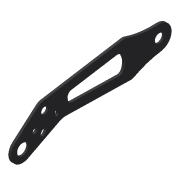
# Autodesk Inventor part: UPPER_LEG_OUTER_FRAME
Saved by Autodesk Inventor 2019.4 (Build 234330000, 330)
## iProperties
Created: 2019-11-12
Part Number: UPPER_LEG_OUTER_FRAME
Material: 一般
Document SubType Name: Modeling
Designer: y6tada
Density: 1 g/cm^3
Appearance: Black 80
Mass: 5.99749 g
Surface Area: 71.6947 cm^2
Volume: 5.99749 cm^3
Author: y6tada
Autodesk Inventor part; units mm, degrees
ref_plane "YZ Plane" through (0, 0, 0) normal (1, 0, 0) x (0, 1, 0)
ref_plane "XZ Plane" through (0, 0, 0) normal (0, 1, 0) x (-1, 0, 0)
ref_plane "XY Plane" through (0, 0, 0) normal (0, 0, 1) x (1, 0, 0)
sketch "スケッチ1" plane through (0, 0, 0) normal (1, 0, 0) x (0, 1, 0)
  line L0 (0, 0) -> (-25, 122.4745) construction
  line L1 (0, 189.3993) -> (0, 0) construction
  line L2 (1.3896, 108.1627) -> (-17.0322, 129.3894)
  arc A0 (-17.0322, 129.3894) -> (-34.3718, 117.6297) centre (-25, 122.4745) ccw
  arc A1 (3.2791, 104.1358) -> (1.3896, 108.1627) centre (-4.7732, 102.8143) ccw
  arc A2 (-17.7874, 128.734) -> (-30.0598, 114.375) centre (-25, 122.4745) ccw construction
  circle A3 centre (-4.7732, 102.8143) radius 7.16 construction
  line L3 (2.2923, 103.9738) -> (18.8479, 3.0931) construction
  line L4 (0.6344, 107.5073) -> (-17.7874, 128.734) construction
  line L5 (-30.0598, 114.375) -> (-18.9414, 107.4293) construction
  line L6 (-16.9441, 103.7364) -> (-19.0959, 0.3976) construction
  arc A4 (-16.9441, 103.7364) -> (-18.9414, 107.4293) centre (-21.1932, 103.8249) ccw construction
  circle A5 centre (-21.1932, 103.8249) radius 4 construction
  arc A6 (-21.8382, 104.2725) -> (-20.5116, 103.4352) centre (-16.3894, 111.4356) ccw construction
  arc A7 (-23.0793, 102.6409) -> (-21.4505, 101.6128) centre (-16.3894, 111.4356) ccw
  arc A8 (-21.4505, 101.6128) -> (-19.5726, 105.2575) centre (-20.5116, 103.4352) ccw
  arc A9 (-20.5971, 105.9041) -> (-23.0793, 102.6409) centre (-21.8382, 104.2725) ccw
  line L7 (-20.5116, 103.4352) -> (-16.3894, 111.4356) construction
  line L8 (-16.3894, 111.4356) -> (-21.8382, 104.2725) construction
  circle A10 centre (-16.3894, 111.4356) radius 2.05
  line L9 (-25, 122.4745) -> (-16.3894, 111.4356) construction
  arc A11 (14.8297, 29.3873) -> (10.9795, 0.6715) centre (85.8396, 5.2502) ccw
  arc A12 (-10.8792, -1.6259) -> (10.9795, 0.6715) centre (0, 0) ccw
  arc A13 (-10.8792, -1.6259) -> (-18.8693, 22.5646) centre (-85.0554, -12.7116) ccw
  line L10 (15.0698, 32.2899) -> (3.2791, 104.1358)
  line L11 (-18.3235, 85.5278) -> (-19.5731, 25.5116)
  line L12 (-16.3894, 111.4356) -> (-21.1932, 103.8249) construction
  arc A14 (-20.5971, 105.9041) -> (-19.5726, 105.2575) centre (-16.3894, 111.4356) ccw
  arc A15 (-13.6957, 91.6178) -> (-10.2953, 92.3867) centre (-16.3894, 111.4356) ccw construction
  line L13 (-10.2953, 92.3867) -> (-16.3894, 111.4356) construction
  line L14 (-13.6957, 91.6178) -> (-16.3894, 111.4356) construction
  arc A16 (-13.8371, 92.6583) -> (-10.6152, 93.3867) centre (-16.3894, 111.4356) ccw
  arc A17 (-13.5542, 90.5774) -> (-9.9753, 91.3866) centre (-16.3894, 111.4356) ccw
  arc A18 (-9.9753, 91.3866) -> (-10.6152, 93.3867) centre (-10.2953, 92.3867) ccw
  arc A19 (-13.8371, 92.6583) -> (-13.5542, 90.5774) centre (-13.6957, 91.6178) ccw
  line L15 (0, 0) -> (-9.0971, 86.5528) construction
  line L16 (-16.3894, 111.4356) -> (-11.9787, 91.928) construction
  arc A20 (-19.0959, 0.3976) -> (18.8479, 3.0931) centre (0, 0) ccw construction
  line L17 (-34.3718, 117.6297) -> (-18.7693, 87.4479)
  arc A21 (-18.3235, 85.5278) -> (-18.7693, 87.4479) centre (-22.3226, 85.611) ccw
  circle A22 centre (-21.1932, 103.8249) radius 5 construction
  arc A23 (14.8297, 29.3873) -> (15.0698, 32.2899) centre (9.149, 31.3183) ccw
  arc A24 (-19.5731, 25.5116) -> (-18.8693, 22.5646) centre (-13.5744, 25.3867) ccw
  circle A25 centre (-21.8382, 104.2725) radius 5 construction
  line L18 (10.9795, 0.6715) -> (0, 0) construction
  line L19 (0, 0) -> (-10.8792, -1.6259) construction
  line L20 (5.3923, 89.8056) -> (-23.9461, 86.722) construction
  line L21 (-15.4306, 104.3676) -> (-17.568, 1.7197) construction
  circle A26 centre (-13.6957, 91.6178) radius 2 construction
  line L22 (6.0142, 38.0699) -> (-0.6771, 78.8428)
  line L23 (-10.4767, 78.0835) -> (-11.3537, 35.9665)
  line L24 (-5.0424, 82.1731) -> (-6.8957, 81.9783)
  circle A27 centre (-3.7775, 43.594) radius 12 construction
  arc A28 (-9.0379, 32.2547) -> (4.8174, 34.5177) centre (-3.7775, 43.594) ccw
  arc A29 (4.8174, 34.5177) -> (6.0142, 38.0699) centre (2.067, 37.4221) ccw
  arc A30 (-11.3537, 35.9665) -> (-9.0379, 32.2547) centre (-7.3546, 35.8833) ccw
  arc A31 (-6.8957, 81.9783) -> (-10.4767, 78.0835) centre (-6.4776, 78.0002) ccw
  arc A32 (-0.6771, 78.8428) -> (-5.0424, 82.1731) centre (-4.6243, 78.195) ccw
  point P0 (19.3766, 87.437)
  point P1 (-18.2579, 88.6771)
  point P2 (15.3178, 30.7783)
  point P3 (-11.4012, 33.6879)
  point P4 (6.3174, 36.2222)
  dimension "d2" = 125
  dimension "d10" = 19.1
  dimension "d11" = 14.32
  dimension "d13" = 8
  dimension "d14" = 0.25
  dimension "d18" = 9
  dimension "d19" = 10
  dimension "d20" = 4.1
  dimension "d25" = 11
  dimension "d35" = 14
  dimension "d40" = 10
  dimension "d41" = 1.05
  dimension "d70" = 45
  dimension "d72" = 20
  dimension "d73" = 2.05
  dimension "d75" = 19.1
  dimension "d76" = 6
  dimension "d77" = 25
  dimension "d78" = 1
  dimension "d79" = 1
  dimension "d80" = 4
  dimension "d81" = 1
  dimension "d82" = 1
  dimension "d84" = 10
  dimension "d86" = 6
  dimension "d87" = 75
  dimension "d88" = 175
  dimension "d90" = 6
  dimension "d91" = 1.5
  dimension "d92" = 4
  dimension "d93" = 14
  dimension "d94" = 8
  dimension "d95" = 8
  dimension "d96" = 4
  dimension "d97" = 0.5
  dimension "d98" = 6.5
  constraints: 61 point on circle, 50 end point, 38 tangent, 33 centre point, 15 coincident, 9 point on line, 5 equal radius, 5 parallel, 3 concentric, 1 symmetric about line, 1 vertical, 5 other
  measures "d2" distance of L0.end L0.start
  measures "d10" diameter of A2
  measures "d11" diameter of A3
  measures "d13" diameter of A5
  measures "d14" radial gap between concentric circles of A5 A4
  measures "d18" radius of A6
  measures "d19" angle of L7 L8
  measures "d20" diameter of A10
  measures "d25" radius of A12
  measures "d35" distance of L0.end L9.end
  measures "d40" angle of L13 L14
  measures "d41" radius of A18
  measures "d70" angle of L12 L16
  measures "d72" radius of A15
  measures "d73" radius of A8
  measures "d75" radius of A20
  measures "d76" angle of L1 L15
  measures "d77" distance from line of A0.centre L1
  measures "d78" distance between parallel lines of L10 L3
  measures "d79" radial gap between concentric circles of A0 A2
  measures "d80" radius of A21
  measures "d81" distance between parallel lines of L11 L6
  measures "d82" radial gap between concentric circles of A5 A22
  measures "d84" diameter of A25
  measures "d86" radius of A23
  measures "d87" radius of A11
  measures "d88" angle of L19 L18
  measures "d90" distance from line of L15 A1.centre
  measures "d91" distance between parallel lines of L6 L21
  measures "d92" diameter of A26
  measures "d93" distance from line of A1.centre L20
  measures "d94" distance between parallel lines of L10 L22
  measures "d95" distance between parallel lines of L11 L23
  measures "d96" radius of A29
  measures "d97" radial gap between concentric circles of A28 A27
  measures "d98" distance between parallel lines of L20 L24
extrude "押し出し1" add sketch "スケッチ1" along normal blind 2
hole "穴1" at (0, 0, 0) direction (1, 0, 0) diameter 8 end through all counterbore diameter 9.3 counterbore depth 0.65
hole "穴2" at (0, -4.7732, 102.8143) direction (1, 0, 0) diameter 6 end through all counterbore diameter 7.3 counterbore depth 0.65
hole "穴3" at (0, -25, 122.4745) direction (1, 0, 0) diameter 10 end through all counterbore diameter 11.3 counterbore depth 0.65
